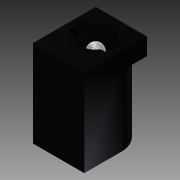
# Autodesk Inventor part: jack
Saved by Autodesk Inventor 2014 SP1 (Build 180222100, 222)
## iProperties
Created: 2014-04-13
Part Number: jack
Material: PET Plastic
Document SubType Name: Modeling
Designer: Tyler
Density: 1.541 g/cm^3
Appearance: Smooth - Black
Author: Tyler
Autodesk Inventor part; units mm, degrees
ref_plane "YZ Plane" through (0, 0, 0) normal (1, 0, 0) x (0, 1, 0)
ref_plane "XZ Plane" through (0, 0, 0) normal (0, 1, 0) x (-1, 0, 0)
ref_plane "XY Plane" through (0, 0, 0) normal (0, 0, 1) x (1, 0, 0)
sketch "Sketch1" plane through (0, 0, 0) normal (0, 0, 1) x (1, 0, 0)
  line L0 (-4.5, 11) -> (4.5, 11)
  line L1 (4.5, 11) -> (4.5, 0)
  line L2 (4.5, 0) -> (-4.5, 0)
  line L3 (-4.5, 0) -> (-4.5, 11)
  point P0 (0, 0)
  dimension "d0" = 9
  dimension "d1" = 0
  dimension "d2" = 11
  dimension "d3" = 4.5
  constraints: 8 end point, 2 parallel, 1 horizontal, 1 perpendicular
  measures "d0" distance of L1.end L2.end
  measures "d1" distance from line of L2 point (0, 0)
  measures "d2" distance of L0.end L1.end
  measures "d3" distance from line of point (0, 0) L1
extrude "Extrusion1" add sketch "Sketch1" against normal blind 15.3
sketch "Sketch2" plane through (0, 0, 0) normal (0, 0, 1) x (1, 0, 0)
  line L0 (4.5, 0) -> (-4.5, 0) projected
  circle A0 centre (0, 6.5) radius 2.85
  point P0 (0, 0)
  dimension "d6" = 5.7
  dimension "d7" = 6.5
  constraints: 1 centre point
  measures "d6" diameter of A0
  measures "d7" distance from line of L0 A0.centre
extrude "Extrusion2" cut sketch "Sketch2" against normal blind 10
sketch "Sketch4" plane through (0, 0, 0) normal (0, 0, 1) x (1, 0, 0)
  circle A0 centre (0, 6.5) radius 2.85 projected
  line L0 (4.5, 11) -> (4.5, 0) projected
  arc A1 (-3.1623, 8) -> (-3.1623, 5) centre (0, 6.5) ccw
  arc A2 (3.1623, 5) -> (3.1623, 8) centre (0, 6.5) ccw
  line L1 (-3.1623, 8) -> (3.1623, 8)
  line L2 (-3.1623, 5) -> (3.1623, 5)
  point P0 (0, 0)
  dimension "d17" = 3.5
  dimension "d18" = 3
  dimension "d19" = 1.5
  constraints: 4 end point, 4 point on circle, 2 centre point, 1 coincident, 1 concentric, 1 parallel, 1 perpendicular
  measures "d17" radius of A2
  measures "d18" distance between parallel lines of L1 L2
  measures "d19" distance from line of A0.centre L1
extrude "Extrusion4" cut sketch "Sketch4" against normal blind 2 contours A0 L2 L1 | A0 L1 A2 L2 | A0 L2 A1 L1
sketch "Sketch3" plane through (0, 6.5, -10) normal (0, 0, 1) x (1, 0, 0)
  circle A0 centre (0, 0) radius 2.85 projected
  circle A1 centre (0, 0) radius 1.25
  point P0 (0, -6.5)
  dimension "d10" = 2.5
  constraints: 1 centre point, 1 coincident
  measures "d10" diameter of A1
extrude "Extrusion3" add sketch "Sketch3" along normal blind 9 contours A1
fillet "Fillet1" radius 1.25 1 edges at (-1.25, 6.5, -1)
sketch "Sketch5" plane through (0, 0, -15.3) normal (0, 0, -1) x (-1, 0, 0)
  line L0 (4.5, 11) -> (-4.5, 11) projected
  line L1 (-4.5, 11) -> (-4.5, 0) projected
  line L2 (-4.5, 0) -> (4.5, 0) projected
  line L3 (4.5, 0) -> (4.5, 11) projected
  arc A0 (4.5, 6.5) -> (-4.5, 6.5) centre (0, 6.5) ccw
  point P0 (0, 0)
  dimension "d22" = 0
  dimension "d23" = 9
  constraints: 2 point on circle, 2 point on line, 1 centre point, 1 tangent
  measures "d22" distance edge to line of A0 L0
  measures "d23" diameter of A0
extrude "Extrusion5" cut sketch "Sketch5" against normal blind 12.3 contours L3 A0 L0 | A0 L1 L0
body "Solid1"
